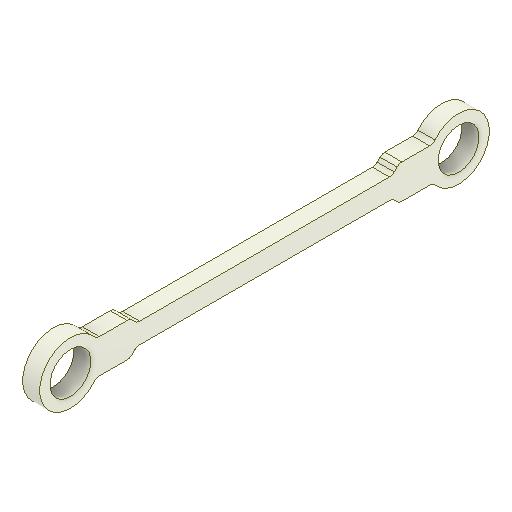
# Autodesk Inventor part: Link_FG
Saved by Autodesk Inventor 2026.2 (Build 302298000, 298)
## iProperties
Created: 2025-12-27
Part Number: Link_FG
Material: 一般
Document SubType Name: Modeling
Designer: Hsiangyu
Density: 1 g/cm^3
Appearance: 平滑 - 象牙白
Author: Hsiangyu
Autodesk Inventor part; units mm, degrees
ref_plane "YZ Plane" through (0, 0, 0) normal (1, 0, 0) x (0, 1, 0)
ref_plane "XZ Plane" through (0, 0, 0) normal (0, 1, 0) x (-1, 0, 0)
ref_plane "XY Plane" through (0, 0, 0) normal (0, 0, 1) x (1, 0, 0)
sketch "草圖1" plane through (0, 0, 0) normal (1, 0, 0) x (0, 1, 0)
  line L0 (0, 0) -> (0, -113.9)
  circle A0 centre (0, 0) radius 6
  circle A1 centre (0, -113.9) radius 6
  circle A2 centre (0, 0) radius 9
  circle A3 centre (0, -113.9) radius 9
  line L1 (5, -7.4833) -> (5, -17.4833)
  line L2 (5, -17.4833) -> (3, -19.4833)
  line L3 (3, -19.4833) -> (3, -94.4167)
  line L4 (3, -94.4167) -> (5, -96.4167)
  line L5 (5, -96.4167) -> (5, -106.4167)
  line L6 (-5, -7.4833) -> (-5, -17.4833)
  line L7 (-5, -17.4833) -> (-3, -19.4833)
  line L8 (-3, -19.4833) -> (-3, -94.4167)
  line L9 (-3, -94.4167) -> (-5, -96.4167)
  line L10 (-5, -96.4167) -> (-5, -106.4167)
  dimension "d0" = 113.9
  dimension "d1" = 12
  dimension "d2" = 12
  dimension "d3" = 18
  dimension "d4" = 18
  dimension "d5" = 3
  dimension "d6" = 3
  dimension "d7" = 135
  dimension "d8" = 5
  dimension "d9" = 10
  dimension "d10" = 10
  dimension "d11" = 135
  constraints: 22 end point, 6 horizontal alignment, 4 centre point, 4 coincident, 4 point on circle, 3 point on line, 3 vertical, 2 parallel
  measures "d0" distance of L0.start L0.end
  measures "d1" diameter of A0
  measures "d2" diameter of A1
  measures "d3" diameter of A2
  measures "d4" diameter of A3
  measures "d5" distance between parallel lines of L0 L3
  measures "d6" distance between parallel lines of L0 L8
  measures "d7" angle of L3 L2
  measures "d8" distance between parallel lines of L0 L1
  measures "d9" distance of L1.start L1.end
  measures "d10" distance of L4.end L5.end
  measures "d11" angle of L3 L4
extrude "擠出1" add sketch "草圖1" along normal mid plane 5
fillet "圓角1" radius 2 12 edges at (0, 5, -7.4833) (0, 5, -17.4833) (0, 3, -19.4833) (0, 3, -94.4167) (0, 5, -96.4167) (0, 5, -106.4167) (0, -5, -7.4833) (0, -5, -17.4833) (0, -3, -19.4833) (0, -3, -94.4167) (0, -5, -96.4167) (0, -5, -106.4167)
equation "\"d2\" = d1"
equation "\"d4\" = d3"
equation "\"d6\" = d5"
equation "\"d10\" = d9"
equation "\"d11\" = d7"
